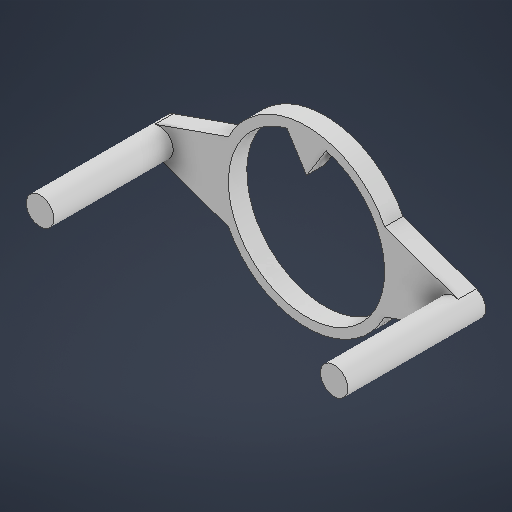
# Autodesk Inventor part: shooter handle
Saved by Autodesk Inventor 2026.2 (Build 302298000, 298)
## iProperties
Created: 2026-03-08
Part Number: shooter handle
Material: Generic
Document SubType Name: Modeling
Designer: danda
Density: 1 g/cm^3
Appearance: Default
Author: danda
Autodesk Inventor part; units mm, degrees
ref_plane "YZ Plane" through (0, 0, 0) normal (1, 0, 0) x (0, 1, 0)
ref_plane "XZ Plane" through (0, 0, 0) normal (0, 1, 0) x (-1, 0, 0)
ref_plane "XY Plane" through (0, 0, 0) normal (0, 0, 1) x (1, 0, 0)
sketch "Sketch1" plane through (0, 0, 0) normal (0, 0, 1) x (1, 0, 0)
  circle A0 centre (85, 85) radius 85
  circle A1 centre (245, 85) radius 15
  line L0 (85, 85) -> (170, 127.4264)
  line L1 (85, 85) -> (170, 42.5736)
  arc A2 (170, 42.5736) -> (170, 127.4264) centre (85, 85) ccw
  line L2 (170, 127.4264) -> (250, 99.1421)
  line L3 (170, 42.5736) -> (250, 70.8579)
  line L4 (85, 85) -> (85, 224.6699)
  line L5 (85, 224.6699) -> (85, -37.035)
  circle A3 centre (-75, 85) radius 15
  line L6 (85, 85) -> (0, 127.4264)
  line L7 (85, 85) -> (0, 42.5736)
  arc A4 (0, 127.4264) -> (0, 42.5736) centre (85, 85) ccw
  line L8 (0, 127.4264) -> (-80, 99.1421)
  line L9 (0, 42.5736) -> (-80, 70.8579)
  circle A5 centre (85, 85) radius 95
  line L10 (63.7027, 167.2887) -> (85, 133.4298)
  line L11 (85, 133.4298) -> (106.2973, 167.2887)
  point P0 (0, 0)
  point P1 (161.0526, 122.9605)
  point P2 (161.0526, 47.0395)
  point P3 (8.9474, 47.0395)
  point P4 (8.9474, 122.9605)
  point P5 (170, 42.5736)
  point P6 (0, 42.5736)
  point P7 (170, 127.4264)
  point P8 (0, 127.4264)
  point P9 (85, 143.723)
  dimension "d0" = 170
  dimension "d1" = 85
  dimension "d2" = 85
  dimension "d3" = 30
  dimension "d5" = 160
  dimension "d12" = 85
  dimension "d14" = 53.051
  dimension "d19" = 40
  dimension "d20" = 32.17
  dimension "d21" = 32.17
  constraints: 24 end point, 10 point on circle, 6 centre point, 5 symmetric about line, 3 point on line, 2 tangent, 1 coincident, 1 vertical, 2 other
  measures "d0" diameter of A0
  measures "d1" horizontal distance of point (0, 0) L0.start
  measures "d2" horizontal distance of point (0, 0) L0.start
  measures "d3" diameter of A1
  measures "d5" distance of L0.start A1.centre
  measures "d12" vertical distance of point (0, 0) A1.centre
  measures "d14" angle of L1 L0
  measures "d19" distance of L10.start L10.end
  measures "d20" angle of L4 L10
  measures "d21" angle of L5 L11
extrude "Extrusion1" add sketch "Sketch1" along normal blind 20 contours A0 L0 A2 L1 | A0 L4 A5 L0 | L1 A5 L5 A0 | L11 L4 A0 | L2 A1 L3 A2 | L5 A5 L7 A0 | L4 L10 A0 | A0 L6 A5 L4 | A0 L7 A4 L6 | A4 L9 A3 L8
extrude "Extrusion2" add sketch "Sketch1" along normal blind 150 contours A1 | A3
body "Solid1"
